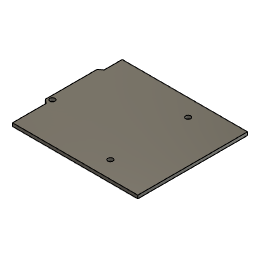
Modular Test Bench - Nucleo v12 (Autodesk Fusion 360 archive; units mm, degrees)
design "Nucleo-L476RG Board"
Autodesk Fusion 360 part; units mm, degrees
sketch "Sketch1" plane through (0, 0, 0) normal (0, 1, 0) x (1, 0, 0)
  line L0 (0, 0) -> (82.5, 0)
  line L1 (82.5, 0) -> (82.5, -70)
  line L2 (82.5, -70) -> (0, -70)
  line L3 (0, -70) -> (0, 0)
  line L4 (2.54, -70) -> (2.54, -48.5)
  line L5 (2.54, -48.5) -> (0, -46.5)
  line L6 (2.54, 0) -> (2.54, -11.5)
  line L7 (2.54, -11.5) -> (0, -13.5)
  dimension "d1" = 82.5
  dimension "d2" = 70
  dimension "d3" = 33
  dimension "d4" = 11.5
  dimension "d5" = 2.54
  dimension "d6" = 2.54
  dimension "d7" = 21.5
  dimension "d8" = 2
  constraint horizontal L0
  constraint vertical L1
  constraint horizontal L2
  constraint vertical L3
  constraint coincident L0.start L3.end
  constraint coincident L2 L4.start
  constraint perpendicular L2 L4
  constraint coincident L3 L5.end
  constraint coincident L0 L6.start
  constraint perpendicular L0 L6
  constraint coincident L3 L7.end
  measures "d1" distance of L1.end L2.end
  measures "d2" distance of L0.start L2.end
  measures "d3" distance of L5.end L7.end
  measures "d4" distance of L6.start L6.end
  measures "d5" distance of L3 L4
  measures "d6" distance of L3 L6
  measures "d7" distance of L4.start L4.end
  measures "d8" vertical distance of L4.end L5.end
extrude "Extrude1" add sketch "Sketch1" along normal blind 2 contours L0 L1 L2 L3 L4 L5 L6 L7
sketch "Sketch2" plane through (0, 2, 0) normal (0, 1, 0) x (-1, 0, 0)
  line L0 (-2.54, 0) -> (-2.54, 11.5)
  line L1 (-2.54, 11.5) -> (0, 13.5)
  line L2 (0, 13.5) -> (0, 46.5)
  line L3 (0, 46.5) -> (-2.54, 48.5)
  line L4 (-2.54, 48.5) -> (-2.54, 70)
  line L5 (-2.54, 70) -> (-82.5, 70)
  line L6 (-82.5, 70) -> (-82.5, 0)
  line L7 (-82.5, 0) -> (-2.54, 0)
  circle A0 centre (-2.54, 44.5) radius 1.6
  circle A1 centre (-54.14, 59.13) radius 1.6
  circle A2 centre (-55.54, 10.87) radius 1.6
  dimension "d11" = 3.2
  dimension "d12" = 2.54
  dimension "d13" = 33
  dimension "d14" = 3.2
  dimension "d15" = 3.2
  dimension "d17" = 10.87
  dimension "d20" = 53
  dimension "d21" = 51.6
  dimension "d22" = 48.26
  measures "d11" diameter of A0
  measures "d12" distance of L2 A0.centre
  measures "d13" distance of L0.end A0.centre
  measures "d14" diameter of A2
  measures "d15" diameter of A1
  measures "d17" distance of L7 A2.centre
  measures "d20" distance of L0 A2.centre
  measures "d21" distance of L4 A1.centre
  measures "d22" vertical distance of A1.centre A2.centre
extrude "Extrude2" cut sketch "Sketch2" against normal blind 2 contours A0 | A1 | A2
